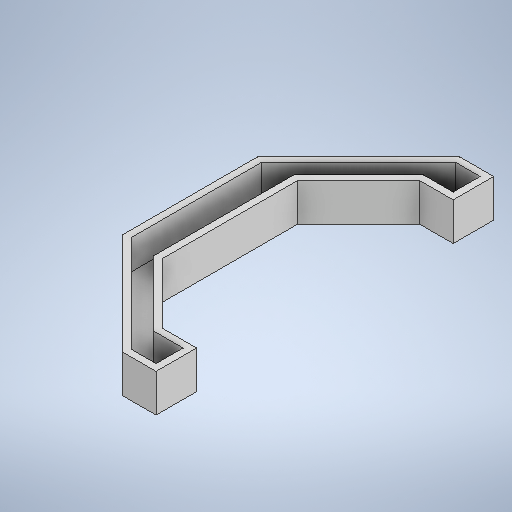
# Autodesk Inventor part: prettylny
Saved by Autodesk Inventor 2025.3 (Build 293356000, 356)
## iProperties
Created: 2026-04-18
Part Number: prettylny
Material: Generic
Document SubType Name: Modeling
Designer: ksawe
Density: 1 g/cm^3
Appearance: Default
Author: ksawe
Autodesk Inventor part; units mm, degrees
ref_plane "YZ Plane" through (0, 0, 0) normal (1, 0, 0) x (0, 1, 0)
ref_plane "XZ Plane" through (0, 0, 0) normal (0, 1, 0) x (-1, 0, 0)
ref_plane "XY Plane" through (0, 0, 0) normal (0, 0, 1) x (1, 0, 0)
sketch "Sketch1" plane through (0, 0, 0) normal (0, 1, 0) x (-1, 0, 0)
  line L0 (-70, 125) -> (-70, 95)
  line L1 (-70, 95) -> (-45, 95)
  line L2 (-45, 95) -> (0, 50)
  line L3 (0, 50) -> (0, 0)
  line L4 (-70, 125) -> (-45, 125)
  line L5 (-45, 125) -> (30, 50)
  line L6 (30, 50) -> (30, 0)
  line L7 (0, 0) -> (-70, 0) construction
  line L8 (-70, -125) -> (-70, -95)
  line L9 (-70, -95) -> (-45, -95)
  line L10 (-45, -95) -> (0, -50)
  line L11 (0, -50) -> (0, 0)
  line L12 (-70, -125) -> (-45, -125)
  line L13 (-45, -125) -> (30, -50)
  line L14 (30, -50) -> (30, 0)
  line L15 (-42.9289, 100) -> (-65, 100)
  line L16 (-65, 100) -> (-65, 120)
  line L17 (-65, 120) -> (-47.0711, 120)
  line L18 (-47.0711, 120) -> (25, 47.9289)
  line L19 (25, 47.9289) -> (25, 0)
  line L20 (25, 0) -> (25, -47.9289)
  line L21 (25, -47.9289) -> (-47.0711, -120)
  line L22 (-47.0711, -120) -> (-65, -120)
  line L23 (-65, -120) -> (-65, -100)
  line L24 (-65, -100) -> (-42.9289, -100)
  line L25 (-42.9289, -100) -> (5, -52.0711)
  line L26 (5, -52.0711) -> (5, 0)
  line L27 (5, 0) -> (5, 52.0711)
  line L28 (5, 52.0711) -> (-42.9289, 100)
  dimension "d0" = 125
  dimension "d1" = 30
  dimension "d4" = 30
  dimension "d5" = 25
  dimension "d6" = 100
  dimension "d7" = 20
  constraints: 58 end point, 6 symmetric about line, 6 vertical alignment, 4 horizontal alignment, 4 parallel, 4 perpendicular, 3 coincident, 1 horizontal, 1 vertical, 13 other
  measures "d0" distance between parallel lines of L7 L4
  measures "d1" distance between parallel lines of L1 L4
  measures "d4" distance between parallel lines of L3 L6
  measures "d5" distance of L0.start L4.end
  measures "d6" distance between parallel lines of L6 L0
  measures "d7" distance between parallel lines of L19 L27
extrude "Extrusion3" add sketch "Sketch1" along normal mid plane 6 contours L4 L5 L6 L14 L13 L12 L8 L9 L10 L11 L3 L2 L1 L0 | L15 L16 L17 L18 L19 L20 L21 L22 L23 L24 L25 L26 L27 L28
extrude "Extrusion4" add sketch "Sketch1" along normal blind 25
sketch "Sketch2" plane through (-30, -3, -50) normal (-1, 0, 0) x (0, 0, 1)
  circle A0 centre (50, 15) radius 6
  point P0 (50, 3)
  dimension "d16" = 12
  constraints: 1 centre point
  measures "d16" diameter of A0
extrude "Extrusion5" add sketch "Sketch2" along normal blind 2
body "Solid2"
